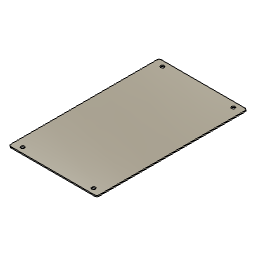
V3 Enclosure BOTTOM v4_FABBED (Autodesk Fusion 360 design; units mm, degrees)
Autodesk Fusion 360 part; units mm, degrees
note: some values were not read from the file. Set by a fixed rule: the direction of a hole.
sketch "Sketch1" plane through (0, 0, 0) normal (0, 0, 1) x (1, 0, 0)
  line L0 (-3, 140) -> (79, 140)
  line L1 (79, 140) -> (79, 0)
  line L2 (79, 0) -> (-3, 0)
  line L3 (-3, 0) -> (-3, 140)
  point P0 (5, 135)
  point P1 (71, 135)
  point P2 (71, 5)
  point P3 (5, 5)
  dimension "d1" = 82
  dimension "d2" = 140
  dimension "d3" = 5
  dimension "d4" = 5
  dimension "d5" = 8
  dimension "d6" = 8
  constraint horizontal L0
  constraint vertical L1
  constraint horizontal L2
  constraint vertical L3
  constraint horizontal P0 P1
  constraint vertical P1 P2
  constraint horizontal P2 P3
  constraint vertical P0 P3
  measures "d1" distance of L0.start L0.end
  measures "d2" distance of L0.start L2.end
  measures "d3" distance of L0 P1
  measures "d4" distance of L2 P2
  measures "d5" distance of L1 P2
  measures "d6" distance of L3 P3
extrude "Face1" add sketch "Sketch1" along normal blind 1.02
hole "Hole1" at (5, 135, 0) at (71, 135, 0) at (71, 5, 0) at (5, 5, 0) direction (0, 0, 1) diameter 3.25 end through all
fillet "Fillet1" radius 2 4 edges at (79, 0, 0.51) (-3, 0, 0.51) (-3, 140, 0.51) (79, 140, 0.51)
